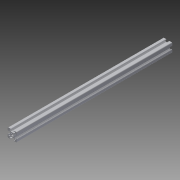
# Autodesk Inventor part: Bosch 20x20 9 in
Saved by Autodesk Inventor 2015 SP1 (Build 190203100, 203)
## iProperties
Created: 2011-07-25
Part Number: Bosch 20x20 9 in
Document SubType Name: Modeling
Designer: Dan Niemitalo
Density: 1 g/cm^3
Material: Aluminum 6061
Appearance: Aluminum - Flat
Author: Dan Niemitalo
Autodesk Inventor part; units mm, degrees
ref_plane "YZ Plane" through (0, 0, 0) normal (1, 0, 0) x (0, 1, 0)
ref_plane "XZ Plane" through (0, 0, 0) normal (0, 1, 0) x (-1, 0, 0)
ref_plane "XY Plane" through (0, 0, 0) normal (0, 0, 1) x (1, 0, 0)
sketch "20x20" plane through (0, 0, 0) normal (0, 0, 1) x (1, 0, 0)
  line L0 (0.5, 16) -> (1.2322, 16)
  arc A0 (1.5858, 15.8536) -> (1.2322, 16) centre (1.2322, 15.5) ccw
  line L1 (2.5, 17.2678) -> (2.5, 18)
  arc A1 (2.5, 17.2678) -> (2.6464, 16.9142) centre (3, 17.2678) ccw
  line L2 (1.5858, 15.8536) -> (3.8536, 13.5858)
  arc A2 (3, 18.5) -> (2.5, 18) centre (3, 18) ccw
  line L3 (4.9142, 14.6464) -> (2.6464, 16.9142)
  line L4 (4.75, 20) -> (0, 20)
  line L5 (3, 18.5) -> (5, 18.5)
  arc A3 (0, 4.5) -> (0.5, 4) centre (0.5, 4.5) ccw
  line L6 (1.2322, 4) -> (0.5, 4)
  arc A4 (1.2322, 4) -> (1.5858, 4.1464) centre (1.2322, 4.5) ccw
  arc A5 (2.6464, 3.0858) -> (2.5, 2.7322) centre (3, 2.7322) ccw
  line L7 (3.8536, 6.4142) -> (1.5858, 4.1464)
  line L8 (2.6464, 3.0858) -> (4.9142, 5.3536)
  arc A6 (5.2678, 5.5) -> (4.9142, 5.3536) centre (5.2678, 5) ccw
  line L9 (2.5, 2) -> (2.5, 2.7322)
  arc A7 (2.5, 2) -> (3, 1.5) centre (3, 2) ccw
  line L10 (0, 0) -> (4.75, 0)
  line L11 (5, 1.5) -> (3, 1.5)
  arc A8 (-1.5, 1.5) -> (0, 0) centre (0, 1.5) ccw
  line L12 (-1.5, 6.25) -> (-1.5, 1.5)
  line L13 (0, 4.5) -> (0, 6.5)
  arc A9 (17, 0) -> (18.5, 1.5) centre (17, 1.5) ccw
  line L14 (18.5, 1.5) -> (18.5, 6.25)
  line L15 (17, 6.5) -> (17, 4.5)
  arc A10 (16.5, 4) -> (17, 4.5) centre (16.5, 4.5) ccw
  line L16 (16.5, 4) -> (15.7678, 4)
  arc A11 (15.4142, 4.1464) -> (15.7678, 4) centre (15.7678, 4.5) ccw
  line L17 (14.5, 2.7322) -> (14.5, 2)
  line L18 (15.4142, 4.1464) -> (13.1464, 6.4142)
  arc A12 (14.5, 2.7322) -> (14.3536, 3.0858) centre (14, 2.7322) ccw
  line L19 (12.0858, 5.3536) -> (14.3536, 3.0858)
  line L20 (12.25, 0) -> (17, 0)
  line L21 (14, 1.5) -> (12, 1.5)
  arc A13 (14, 1.5) -> (14.5, 2) centre (14, 2) ccw
  line L22 (17, 20) -> (12.25, 20)
  line L23 (15.7678, 16) -> (16.5, 16)
  arc A14 (14.5, 18) -> (14, 18.5) centre (14, 18) ccw
  arc A15 (17, 15.5) -> (16.5, 16) centre (16.5, 15.5) ccw
  arc A16 (14.3536, 16.9142) -> (14.5, 17.2678) centre (14, 17.2678) ccw
  arc A17 (15.7678, 16) -> (15.4142, 15.8536) centre (15.7678, 15.5) ccw
  line L24 (18.5, 13.75) -> (18.5, 18.5)
  arc A18 (18.3, 13.55) -> (18.5, 13.75) centre (18.3, 13.75) ccw
  line L25 (17, 15.5) -> (17, 13.5)
  line L26 (13.1464, 13.5858) -> (15.4142, 15.8536)
  arc A19 (13.1464, 13.5858) -> (13, 13.2322) centre (13.5, 13.2322) ccw
  line L27 (14.3536, 16.9142) -> (12.0858, 14.6464)
  line L28 (14.5, 18) -> (14.5, 17.2678)
  arc A20 (18.5, 18.5) -> (17, 20) centre (17, 18.5) ccw
  line L29 (12, 18.5) -> (14, 18.5)
  arc A21 (0, 20) -> (-1.5, 18.5) centre (0, 18.5) ccw
  arc A22 (0.5, 16) -> (0, 15.5) centre (0.5, 15.5) ccw
  line L30 (-1.5, 18.5) -> (-1.5, 13.75)
  line L31 (0, 13.5) -> (0, 15.5)
  line L32 (13, 6.7678) -> (13, 9.0464)
  line L33 (11.4922, 8.0901) -> (10.9453, 8.7418)
  arc A23 (10.4139, 7.0104) -> (11.4922, 8.0901) centre (8.5, 10) ccw
  line L34 (9.7582, 7.5547) -> (10.4139, 7.0104)
  arc A24 (7.2418, 7.5547) -> (9.7582, 7.5547) centre (8.5, 10) ccw
  arc A25 (3.8536, 6.4142) -> (4, 6.7678) centre (3.5, 6.7678) ccw
  line L35 (4, 9.0464) -> (4, 6.7678)
  arc A26 (4.0268, 9.1464) -> (4, 9.0464) centre (4.2, 9.0464) ccw
  line L36 (4.4619, 9.9) -> (4.0268, 9.1464)
  arc A27 (4.4619, 9.9) -> (4.4619, 10.1) centre (4.2887, 10) ccw
  arc A28 (4, 10.9536) -> (4.0268, 10.8536) centre (4.2, 10.9536) ccw
  line L37 (4.0268, 10.8536) -> (4.4619, 10.1)
  line L38 (6.0547, 8.7418) -> (5.5078, 8.0901)
  line L39 (5.2678, 5.5) -> (7.5464, 5.5)
  arc A29 (5.5078, 8.0901) -> (6.5861, 7.0104) centre (8.5, 10) ccw
  line L40 (6.5861, 7.0104) -> (7.2418, 7.5547)
  arc A30 (6.0547, 11.2582) -> (6.0547, 8.7418) centre (8.5, 10) ccw
  line L41 (5.5078, 11.9099) -> (6.0547, 11.2582)
  arc A31 (-1.5, 13.75) -> (-1.3, 13.55) centre (-1.3, 13.75) ccw
  line L42 (-1.3, 13.55) -> (-1.2, 13.55)
  arc A32 (-1, 13.35) -> (-1.2, 13.55) centre (-1.2, 13.35) ccw
  arc A33 (-0.5, 13) -> (0, 13.5) centre (-0.5, 13.5) ccw
  line L43 (-1, 13.35) -> (-1, 13.2)
  line L44 (-0.8, 13) -> (-0.5, 13)
  arc A34 (-1, 13.2) -> (-0.8, 13) centre (-0.8, 13.2) ccw
  arc A35 (4.9142, 14.6464) -> (5.2678, 14.5) centre (5.2678, 15) ccw
  arc A36 (4, 13.2322) -> (3.8536, 13.5858) centre (3.5, 13.2322) ccw
  line L45 (7.5464, 14.5) -> (5.2678, 14.5)
  arc A37 (7.6464, 14.4732) -> (7.5464, 14.5) centre (7.5464, 14.3) ccw
  line L46 (7.2418, 12.4453) -> (6.5861, 12.9896)
  line L47 (8.4, 14.0381) -> (7.6464, 14.4732)
  arc A38 (8.4, 14.0381) -> (8.6, 14.0381) centre (8.5, 14.2113) ccw
  line L48 (9.3536, 14.4732) -> (8.6, 14.0381)
  arc A39 (9.4536, 14.5) -> (9.3536, 14.4732) centre (9.4536, 14.3) ccw
  arc A40 (0, 6.5) -> (-0.5, 7) centre (-0.5, 6.5) ccw
  line L49 (-0.5, 7) -> (-0.8, 7)
  arc A41 (-0.8, 7) -> (-1, 6.8) centre (-0.8, 6.8) ccw
  line L50 (-1, 6.8) -> (-1, 6.65)
  arc A42 (-1.2, 6.45) -> (-1, 6.65) centre (-1.2, 6.65) ccw
  line L51 (-1.2, 6.45) -> (-1.3, 6.45)
  arc A43 (-1.3, 6.45) -> (-1.5, 6.25) centre (-1.3, 6.25) ccw
  line L52 (4.95, 0.2) -> (4.95, 0.3)
  arc A44 (5.15, 0.5) -> (4.95, 0.3) centre (5.15, 0.3) ccw
  line L53 (5.15, 0.5) -> (5.3, 0.5)
  arc A45 (5.5, 1) -> (5, 1.5) centre (5, 1) ccw
  arc A46 (4.75, 0) -> (4.95, 0.2) centre (4.75, 0.2) ccw
  arc A47 (5.3, 0.5) -> (5.5, 0.7) centre (5.3, 0.7) ccw
  line L54 (5.5, 0.7) -> (5.5, 1)
  arc A48 (7.5464, 5.5) -> (7.6464, 5.5268) centre (7.5464, 5.7) ccw
  line L55 (7.6464, 5.5268) -> (8.4, 5.9619)
  arc A49 (8.6, 5.9619) -> (8.4, 5.9619) centre (8.5, 5.7887) ccw
  line L56 (8.6, 5.9619) -> (9.3536, 5.5268)
  arc A50 (9.3536, 5.5268) -> (9.4536, 5.5) centre (9.4536, 5.7) ccw
  line L57 (9.4536, 5.5) -> (11.7322, 5.5)
  arc A51 (13, 6.7678) -> (13.1464, 6.4142) centre (13.5, 6.7678) ccw
  arc A52 (12.0858, 5.3536) -> (11.7322, 5.5) centre (11.7322, 5) ccw
  arc A53 (12, 1.5) -> (11.5, 1) centre (12, 1) ccw
  line L58 (12.05, 0.3) -> (12.05, 0.2)
  line L59 (11.7, 0.5) -> (11.85, 0.5)
  arc A54 (12.05, 0.3) -> (11.85, 0.5) centre (11.85, 0.3) ccw
  arc A55 (12.05, 0.2) -> (12.25, 0) centre (12.25, 0.2) ccw
  arc A56 (11.5, 0.7) -> (11.7, 0.5) centre (11.7, 0.7) ccw
  line L60 (11.5, 1) -> (11.5, 0.7)
  arc A57 (17.5, 7) -> (17, 6.5) centre (17.5, 6.5) ccw
  line L61 (18.3, 6.45) -> (18.2, 6.45)
  line L62 (17.8, 7) -> (17.5, 7)
  line L63 (18, 6.65) -> (18, 6.8)
  arc A58 (18, 6.65) -> (18.2, 6.45) centre (18.2, 6.65) ccw
  arc A59 (18, 6.8) -> (17.8, 7) centre (17.8, 6.8) ccw
  arc A60 (18.5, 6.25) -> (18.3, 6.45) centre (18.3, 6.25) ccw
  arc A61 (10.9453, 8.7418) -> (10.9453, 11.2582) centre (8.5, 10) ccw
  arc A62 (13, 9.0464) -> (12.9732, 9.1464) centre (12.8, 9.0464) ccw
  line L64 (12.9732, 9.1464) -> (12.5381, 9.9)
  line L65 (10.4139, 12.9896) -> (9.7582, 12.4453)
  line L66 (10.9453, 11.2582) -> (11.4922, 11.9099)
  arc A63 (11.4922, 11.9099) -> (10.4139, 12.9896) centre (8.5, 10) ccw
  line L67 (12.5381, 10.1) -> (12.9732, 10.8536)
  arc A64 (12.9732, 10.8536) -> (13, 10.9536) centre (12.8, 10.9536) ccw
  line L68 (13, 10.9536) -> (13, 13.2322)
  arc A65 (12.5381, 10.1) -> (12.5381, 9.9) centre (12.7113, 10) ccw
  arc A66 (18.2, 13.55) -> (18, 13.35) centre (18.2, 13.35) ccw
  line L69 (18.2, 13.55) -> (18.3, 13.55)
  line L70 (18, 13.2) -> (18, 13.35)
  arc A67 (17, 13.5) -> (17.5, 13) centre (17.5, 13.5) ccw
  line L71 (17.5, 13) -> (17.8, 13)
  arc A68 (17.8, 13) -> (18, 13.2) centre (17.8, 13.2) ccw
  line L72 (4, 13.2322) -> (4, 10.9536)
  arc A69 (6.5861, 12.9896) -> (5.5078, 11.9099) centre (8.5, 10) ccw
  arc A70 (11.7322, 14.5) -> (12.0858, 14.6464) centre (11.7322, 15) ccw
  line L73 (11.7322, 14.5) -> (9.4536, 14.5)
  arc A71 (9.7582, 12.4453) -> (7.2418, 12.4453) centre (8.5, 10) ccw
  arc A72 (11.5, 19) -> (12, 18.5) centre (12, 19) ccw
  line L74 (11.5, 19.3) -> (11.5, 19)
  line L75 (11.85, 19.5) -> (11.7, 19.5)
  arc A73 (11.85, 19.5) -> (12.05, 19.7) centre (11.85, 19.7) ccw
  arc A74 (12.25, 20) -> (12.05, 19.8) centre (12.25, 19.8) ccw
  arc A75 (11.7, 19.5) -> (11.5, 19.3) centre (11.7, 19.3) ccw
  line L76 (12.05, 19.8) -> (12.05, 19.7)
  arc A76 (5, 18.5) -> (5.5, 19) centre (5, 19) ccw
  line L77 (4.95, 19.7) -> (4.95, 19.8)
  line L78 (5.5, 19) -> (5.5, 19.3)
  line L79 (5.3, 19.5) -> (5.15, 19.5)
  arc A77 (4.95, 19.7) -> (5.15, 19.5) centre (5.15, 19.7) ccw
  arc A78 (4.95, 19.8) -> (4.75, 20) centre (4.75, 19.8) ccw
  arc A79 (5.5, 19.3) -> (5.3, 19.5) centre (5.3, 19.3) ccw
  point P0 (8.5, 10)
sketch "Sketch1" plane through (0, 0, 0) normal (0, 0, 1) x (1, 0, 0)
  line L0 (-8, 6) -> (-7.2678, 6)
  arc A0 (-6.9142, 5.8536) -> (-7.2678, 6) centre (-7.2678, 5.5) ccw
  line L1 (-6, 7.2678) -> (-6, 8)
  arc A1 (-6, 7.2678) -> (-5.8536, 6.9142) centre (-5.5, 7.2678) ccw
  line L2 (-6.9142, 5.8536) -> (-4.6464, 3.5858)
  arc A2 (-5.5, 8.5) -> (-6, 8) centre (-5.5, 8) ccw
  line L3 (-3.5858, 4.6464) -> (-5.8536, 6.9142)
  line L4 (-3.75, 10) -> (-8.5, 10)
  line L5 (-5.5, 8.5) -> (-3.5, 8.5)
  arc A3 (-8.5, -5.5) -> (-8, -6) centre (-8, -5.5) ccw
  line L6 (-7.2678, -6) -> (-8, -6)
  arc A4 (-7.2678, -6) -> (-6.9142, -5.8536) centre (-7.2678, -5.5) ccw
  arc A5 (-5.8536, -6.9142) -> (-6, -7.2678) centre (-5.5, -7.2678) ccw
  line L7 (-4.6464, -3.5858) -> (-6.9142, -5.8536)
  line L8 (-5.8536, -6.9142) -> (-3.5858, -4.6464)
  arc A6 (-3.2322, -4.5) -> (-3.5858, -4.6464) centre (-3.2322, -5) ccw
  line L9 (-6, -8) -> (-6, -7.2678)
  arc A7 (-6, -8) -> (-5.5, -8.5) centre (-5.5, -8) ccw
  line L10 (-8.5, -10) -> (-3.75, -10)
  line L11 (-3.5, -8.5) -> (-5.5, -8.5)
  arc A8 (-10, -8.5) -> (-8.5, -10) centre (-8.5, -8.5) ccw
  line L12 (-10, -3.75) -> (-10, -8.5)
  line L13 (-8.5, -5.5) -> (-8.5, -3.5)
  arc A9 (8.5, -10) -> (10, -8.5) centre (8.5, -8.5) ccw
  line L14 (10, -8.5) -> (10, -3.75)
  line L15 (8.5, -3.5) -> (8.5, -5.5)
  arc A10 (8, -6) -> (8.5, -5.5) centre (8, -5.5) ccw
  line L16 (8, -6) -> (7.2678, -6)
  arc A11 (6.9142, -5.8536) -> (7.2678, -6) centre (7.2678, -5.5) ccw
  line L17 (6, -7.2678) -> (6, -8)
  line L18 (6.9142, -5.8536) -> (4.6464, -3.5858)
  arc A12 (6, -7.2678) -> (5.8536, -6.9142) centre (5.5, -7.2678) ccw
  line L19 (3.5858, -4.6464) -> (5.8536, -6.9142)
  line L20 (3.75, -10) -> (8.5, -10)
  line L21 (5.5, -8.5) -> (3.5, -8.5)
  arc A13 (5.5, -8.5) -> (6, -8) centre (5.5, -8) ccw
  line L22 (8.5, 10) -> (3.75, 10)
  line L23 (7.2678, 6) -> (8, 6)
  arc A14 (6, 8) -> (5.5, 8.5) centre (5.5, 8) ccw
  arc A15 (8.5, 5.5) -> (8, 6) centre (8, 5.5) ccw
  arc A16 (5.8536, 6.9142) -> (6, 7.2678) centre (5.5, 7.2678) ccw
  arc A17 (7.2678, 6) -> (6.9142, 5.8536) centre (7.2678, 5.5) ccw
  line L24 (10, 3.75) -> (10, 8.5)
  arc A18 (9.8, 3.55) -> (10, 3.75) centre (9.8, 3.75) ccw
  line L25 (8.5, 5.5) -> (8.5, 3.5)
  line L26 (4.6464, 3.5858) -> (6.9142, 5.8536)
  arc A19 (4.6464, 3.5858) -> (4.5, 3.2322) centre (5, 3.2322) ccw
  line L27 (5.8536, 6.9142) -> (3.5858, 4.6464)
  line L28 (6, 8) -> (6, 7.2678)
  arc A20 (10, 8.5) -> (8.5, 10) centre (8.5, 8.5) ccw
  line L29 (3.5, 8.5) -> (5.5, 8.5)
  arc A21 (-8.5, 10) -> (-10, 8.5) centre (-8.5, 8.5) ccw
  arc A22 (-8, 6) -> (-8.5, 5.5) centre (-8, 5.5) ccw
  line L30 (-10, 8.5) -> (-10, 3.75)
  line L31 (-8.5, 3.5) -> (-8.5, 5.5)
  line L32 (4.5, -3.2322) -> (4.5, -0.9536)
  line L33 (2.9922, -1.9099) -> (2.4453, -1.2582)
  arc A23 (1.9139, -2.9896) -> (2.9922, -1.9099) centre (0, 0) ccw
  line L34 (1.2582, -2.4453) -> (1.9139, -2.9896)
  arc A24 (-1.2582, -2.4453) -> (1.2582, -2.4453) centre (0, 0) ccw
  arc A25 (-4.6464, -3.5858) -> (-4.5, -3.2322) centre (-5, -3.2322) ccw
  line L35 (-4.5, -0.9536) -> (-4.5, -3.2322)
  arc A26 (-4.4732, -0.8536) -> (-4.5, -0.9536) centre (-4.3, -0.9536) ccw
  line L36 (-4.0381, -0.1) -> (-4.4732, -0.8536)
  arc A27 (-4.0381, -0.1) -> (-4.0381, 0.1) centre (-4.2113, 0) ccw
  arc A28 (-4.5, 0.9536) -> (-4.4732, 0.8536) centre (-4.3, 0.9536) ccw
  line L37 (-4.4732, 0.8536) -> (-4.0381, 0.1)
  line L38 (-2.4453, -1.2582) -> (-2.9922, -1.9099)
  line L39 (-3.2322, -4.5) -> (-0.9536, -4.5)
  arc A29 (-2.9922, -1.9099) -> (-1.9139, -2.9896) centre (0, 0) ccw
  line L40 (-1.9139, -2.9896) -> (-1.2582, -2.4453)
  arc A30 (-2.4453, 1.2582) -> (-2.4453, -1.2582) centre (0, 0) ccw
  line L41 (-2.9922, 1.9099) -> (-2.4453, 1.2582)
  arc A31 (-10, 3.75) -> (-9.8, 3.55) centre (-9.8, 3.75) ccw
  line L42 (-9.8, 3.55) -> (-9.7, 3.55)
  arc A32 (-9.5, 3.35) -> (-9.7, 3.55) centre (-9.7, 3.35) ccw
  arc A33 (-9, 3) -> (-8.5, 3.5) centre (-9, 3.5) ccw
  line L43 (-9.5, 3.35) -> (-9.5, 3.2)
  line L44 (-9.3, 3) -> (-9, 3)
  arc A34 (-9.5, 3.2) -> (-9.3, 3) centre (-9.3, 3.2) ccw
  arc A35 (-3.5858, 4.6464) -> (-3.2322, 4.5) centre (-3.2322, 5) ccw
  arc A36 (-4.5, 3.2322) -> (-4.6464, 3.5858) centre (-5, 3.2322) ccw
  line L45 (-0.9536, 4.5) -> (-3.2322, 4.5)
  arc A37 (-0.8536, 4.4732) -> (-0.9536, 4.5) centre (-0.9536, 4.3) ccw
  line L46 (-1.2582, 2.4453) -> (-1.9139, 2.9896)
  line L47 (-0.1, 4.0381) -> (-0.8536, 4.4732)
  arc A38 (-0.1, 4.0381) -> (0.1, 4.0381) centre (0, 4.2113) ccw
  line L48 (0.8536, 4.4732) -> (0.1, 4.0381)
  arc A39 (0.9536, 4.5) -> (0.8536, 4.4732) centre (0.9536, 4.3) ccw
  arc A40 (-8.5, -3.5) -> (-9, -3) centre (-9, -3.5) ccw
  line L49 (-9, -3) -> (-9.3, -3)
  arc A41 (-9.3, -3) -> (-9.5, -3.2) centre (-9.3, -3.2) ccw
  line L50 (-9.5, -3.2) -> (-9.5, -3.35)
  arc A42 (-9.7, -3.55) -> (-9.5, -3.35) centre (-9.7, -3.35) ccw
  line L51 (-9.7, -3.55) -> (-9.8, -3.55)
  arc A43 (-9.8, -3.55) -> (-10, -3.75) centre (-9.8, -3.75) ccw
  line L52 (-3.55, -9.8) -> (-3.55, -9.7)
  arc A44 (-3.35, -9.5) -> (-3.55, -9.7) centre (-3.35, -9.7) ccw
  line L53 (-3.35, -9.5) -> (-3.2, -9.5)
  arc A45 (-3, -9) -> (-3.5, -8.5) centre (-3.5, -9) ccw
  arc A46 (-3.75, -10) -> (-3.55, -9.8) centre (-3.75, -9.8) ccw
  arc A47 (-3.2, -9.5) -> (-3, -9.3) centre (-3.2, -9.3) ccw
  line L54 (-3, -9.3) -> (-3, -9)
  arc A48 (-0.9536, -4.5) -> (-0.8536, -4.4732) centre (-0.9536, -4.3) ccw
  line L55 (-0.8536, -4.4732) -> (-0.1, -4.0381)
  arc A49 (0.1, -4.0381) -> (-0.1, -4.0381) centre (0, -4.2113) ccw
  line L56 (0.1, -4.0381) -> (0.8536, -4.4732)
  arc A50 (0.8536, -4.4732) -> (0.9536, -4.5) centre (0.9536, -4.3) ccw
  line L57 (0.9536, -4.5) -> (3.2322, -4.5)
  arc A51 (4.5, -3.2322) -> (4.6464, -3.5858) centre (5, -3.2322) ccw
  arc A52 (3.5858, -4.6464) -> (3.2322, -4.5) centre (3.2322, -5) ccw
  arc A53 (3.5, -8.5) -> (3, -9) centre (3.5, -9) ccw
  line L58 (3.55, -9.7) -> (3.55, -9.8)
  line L59 (3.2, -9.5) -> (3.35, -9.5)
  arc A54 (3.55, -9.7) -> (3.35, -9.5) centre (3.35, -9.7) ccw
  arc A55 (3.55, -9.8) -> (3.75, -10) centre (3.75, -9.8) ccw
  arc A56 (3, -9.3) -> (3.2, -9.5) centre (3.2, -9.3) ccw
  line L60 (3, -9) -> (3, -9.3)
  arc A57 (9, -3) -> (8.5, -3.5) centre (9, -3.5) ccw
  line L61 (9.8, -3.55) -> (9.7, -3.55)
  line L62 (9.3, -3) -> (9, -3)
  line L63 (9.5, -3.35) -> (9.5, -3.2)
  arc A58 (9.5, -3.35) -> (9.7, -3.55) centre (9.7, -3.35) ccw
  arc A59 (9.5, -3.2) -> (9.3, -3) centre (9.3, -3.2) ccw
  arc A60 (10, -3.75) -> (9.8, -3.55) centre (9.8, -3.75) ccw
  arc A61 (2.4453, -1.2582) -> (2.4453, 1.2582) centre (0, 0) ccw
  arc A62 (4.5, -0.9536) -> (4.4732, -0.8536) centre (4.3, -0.9536) ccw
  line L64 (4.4732, -0.8536) -> (4.0381, -0.1)
  line L65 (1.9139, 2.9896) -> (1.2582, 2.4453)
  line L66 (2.4453, 1.2582) -> (2.9922, 1.9099)
  arc A63 (2.9922, 1.9099) -> (1.9139, 2.9896) centre (0, 0) ccw
  line L67 (4.0381, 0.1) -> (4.4732, 0.8536)
  arc A64 (4.4732, 0.8536) -> (4.5, 0.9536) centre (4.3, 0.9536) ccw
  line L68 (4.5, 0.9536) -> (4.5, 3.2322)
  arc A65 (4.0381, 0.1) -> (4.0381, -0.1) centre (4.2113, 0) ccw
  arc A66 (9.7, 3.55) -> (9.5, 3.35) centre (9.7, 3.35) ccw
  line L69 (9.7, 3.55) -> (9.8, 3.55)
  line L70 (9.5, 3.2) -> (9.5, 3.35)
  arc A67 (8.5, 3.5) -> (9, 3) centre (9, 3.5) ccw
  line L71 (9, 3) -> (9.3, 3)
  arc A68 (9.3, 3) -> (9.5, 3.2) centre (9.3, 3.2) ccw
  line L72 (-4.5, 3.2322) -> (-4.5, 0.9536)
  arc A69 (-1.9139, 2.9896) -> (-2.9922, 1.9099) centre (0, 0) ccw
  arc A70 (3.2322, 4.5) -> (3.5858, 4.6464) centre (3.2322, 5) ccw
  line L73 (3.2322, 4.5) -> (0.9536, 4.5)
  arc A71 (1.2582, 2.4453) -> (-1.2582, 2.4453) centre (0, 0) ccw
  arc A72 (3, 9) -> (3.5, 8.5) centre (3.5, 9) ccw
  line L74 (3, 9.3) -> (3, 9)
  line L75 (3.35, 9.5) -> (3.2, 9.5)
  arc A73 (3.35, 9.5) -> (3.55, 9.7) centre (3.35, 9.7) ccw
  arc A74 (3.75, 10) -> (3.55, 9.8) centre (3.75, 9.8) ccw
  arc A75 (3.2, 9.5) -> (3, 9.3) centre (3.2, 9.3) ccw
  line L76 (3.55, 9.8) -> (3.55, 9.7)
  arc A76 (-3.5, 8.5) -> (-3, 9) centre (-3.5, 9) ccw
  line L77 (-3.55, 9.7) -> (-3.55, 9.8)
  line L78 (-3, 9) -> (-3, 9.3)
  line L79 (-3.2, 9.5) -> (-3.35, 9.5)
  arc A77 (-3.55, 9.7) -> (-3.35, 9.5) centre (-3.35, 9.7) ccw
  arc A78 (-3.55, 9.8) -> (-3.75, 10) centre (-3.75, 9.8) ccw
  arc A79 (-3, 9.3) -> (-3.2, 9.5) centre (-3.2, 9.3) ccw
  constraints: 1 other
extrude "Extrusion1" add sketch "Sketch1" along normal mid plane 349.25
body "Solid1"
